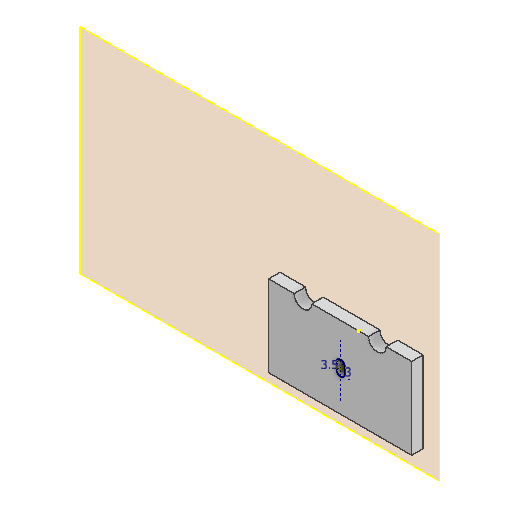
# Autodesk Inventor part: Cuvette Aligner 50mm
Saved by Autodesk Inventor 2025.1 (Build 291241020, 241B)
## iProperties
Created: 2024-09-23
Part Number: Cuvette Aligner 50mm
Material: Generic
Document SubType Name: Modeling
Designer: wayneslade
Density: 1 g/cm^3
Appearance: Default
Author: wayneslade
Autodesk Inventor part; units mm, degrees
ref_plane "YZ Plane" through (0, 0, 0) normal (1, 0, 0) x (0, 1, 0)
ref_plane "XZ Plane" through (0, 0, 0) normal (0, 1, 0) x (-1, 0, 0)
ref_plane "XY Plane" through (0, 0, 0) normal (0, 0, 1) x (1, 0, 0)
ref_plane "Work Plane1" through (0, 0, 0) normal (0, 0, 1) x (1, 0, 0)
sketch "Sketch1" plane through (0, 0, 0) normal (0, 0, 1) x (1, 0, 0)
  circle A0 centre (11.5562, -18) radius 2 construction
  line L0 (-53.1938, -16) -> (-53.1938, -30) construction
  arc A1 (-56.1938, -30) -> (-53.1938, -30) centre (-54.6938, -30) ccw construction
  line L1 (-56.1938, -30) -> (-56.1938, -16) construction
  arc A2 (-53.1938, -16) -> (-56.1938, -16) centre (-54.6938, -16) ccw construction
  line L2 (7.0562, -16) -> (7.0562, -30) construction
  arc A3 (4.0562, -30) -> (7.0562, -30) centre (5.5562, -30) ccw construction
  line L3 (4.0562, -30) -> (4.0562, -16) construction
  arc A4 (7.0562, -16) -> (4.0562, -16) centre (5.5562, -16) ccw construction
  line L4 (-13.1938, -16) -> (-13.1938, -30) construction
  arc A5 (-16.1938, -30) -> (-13.1938, -30) centre (-14.6938, -30) ccw construction
  line L5 (-16.1938, -30) -> (-16.1938, -16) construction
  arc A6 (-13.1938, -16) -> (-16.1938, -16) centre (-14.6938, -16) ccw construction
  arc A7 (19.0562, -16) -> (16.0562, -16) centre (17.5562, -16) ccw construction
  line L6 (19.0562, -16) -> (19.0562, -30) construction
  arc A8 (16.0562, -30) -> (19.0562, -30) centre (17.5562, -30) ccw construction
  line L7 (16.0562, -30) -> (16.0562, -16) construction
  line L8 (22.8064, -40) -> (22.8064, 45) construction
  line L9 (22.8064, 45) -> (-120, 45) construction
  line L10 (-120, 27.5563) -> (-120, 45) construction
  line L11 (-120, 27.5563) -> (-95.2035, 27.5563) construction
  arc A9 (-85.0841, 27.5563) -> (-95.2035, 27.5563) centre (-90.1438, 25.4) ccw construction
  line L12 (-85.0841, 27.5563) -> (17.8062, 27.5563) construction
  line L13 (17.8062, 27.5563) -> (17.8062, -11) construction
  line L14 (17.8062, -11) -> (-120, -11) construction
  line L15 (-120, -40) -> (-120, -11) construction
  line L16 (22.8064, -40) -> (-120, -40) construction
  circle A10 centre (-111.1938, -18) radius 2 construction
  circle A11 centre (-98.1938, -18) radius 2 construction
  circle A12 centre (-61.1938, -18) radius 2 construction
  circle A13 centre (-48.1938, -18) radius 2 construction
  circle A14 centre (-21.1938, -18) radius 2 construction
  circle A15 centre (-8.1938, -18) radius 2 construction
  circle A16 centre (-21.1938, 33.6563) radius 2 construction
  circle A17 centre (-8.1938, 33.6563) radius 2 construction
  circle A18 centre (-61.1938, 33.6563) radius 2 construction
  circle A19 centre (-48.1938, 33.6563) radius 2 construction
  circle A20 centre (-111.1938, 33.6563) radius 2 construction
  circle A21 centre (-98.1938, 33.6563) radius 2 construction
  circle A22 centre (-90.1438, -25.4) radius 5.5 construction
  circle A23 centre (7.8062, 0) radius 3.75 construction
  circle A24 centre (-24.6938, 0) radius 3.75 construction
  line L17 (22.8064, -35.5) -> (-39.6938, -35.5)
  line L18 (-39.6938, -35.5) -> (-39.6938, 0)
  line L19 (-39.6938, 0) -> (-28.5438, 0)
  line L20 (22.8064, 0) -> (22.8064, -35.5)
  line L21 (-34.6938, -11) -> (-34.6938, 11) construction
  arc A25 (3.9562, 0) -> (11.6562, 0) centre (7.8062, 0) ccw
  line L22 (11.6562, 0) -> (22.8064, 0)
  arc A26 (-28.5438, 0) -> (-20.8438, 0) centre (-24.6938, 0) ccw
  line L23 (-20.8438, 0) -> (3.9562, 0)
  point P0 (0, 0)
  point P1 (17.5562, -31.5)
  dimension "d0" = 5
  dimension "d1" = 0
  dimension "d2" = 0.1
  dimension "d3" = 0.1
  dimension "d4" = 4
  constraints: 12 end point, 5 point on circle, 4 parallel, 2 centre point, 2 coincident, 1 horizontal, 1 perpendicular, 1 point on line
  measures "d0" distance between parallel lines of L18 L21
  measures "d1" distance between parallel lines of L20 L8
  measures "d2" radial gap between concentric circles of A23 A25
  measures "d3" radial gap between concentric circles of A24 A26
  measures "d4" distance from line of L17 point (17.556, -31.5)
extrude "Main Body" add sketch "Sketch1" along normal blind 5
sketch "Sketch2" plane through (0, 0, 0) normal (0, 0, -1) x (-1, 0, 0)
  line L0 (16.1938, -30) -> (16.1938, -16) construction
  arc A0 (13.1938, -30) -> (16.1938, -30) centre (14.6938, -30) ccw construction
  line L1 (13.1938, -16) -> (13.1938, -30) construction
  arc A1 (16.1938, -16) -> (13.1938, -16) centre (14.6938, -16) ccw construction
  line L2 (16.1938, -30) -> (16.1938, -16) construction
  line L3 (-4.0562, -30) -> (-4.0562, -16) construction
  arc A2 (-7.0562, -30) -> (-4.0562, -30) centre (-5.5562, -30) ccw construction
  line L4 (-7.0562, -16) -> (-7.0562, -30) construction
  arc A3 (-4.0562, -16) -> (-7.0562, -16) centre (-5.5562, -16) ccw construction
  line L5 (-5.5562, -16) -> (-5.5562, -30) construction
  line L6 (14.6938, -16) -> (14.6938, -30) construction
  line L7 (-5.5562, -17) -> (-5.5562, -29) construction
  line L8 (-7.0062, -17) -> (-7.0062, -29)
  line L9 (-4.1062, -29) -> (-4.1062, -17)
  arc A4 (-4.1062, -17) -> (-7.0062, -17) centre (-5.5562, -17) ccw
  arc A5 (-7.0062, -29) -> (-4.1062, -29) centre (-5.5562, -29) ccw
  line L10 (14.6938, -17) -> (14.6938, -29) construction
  line L11 (13.2438, -17) -> (13.2438, -29)
  line L12 (16.1438, -29) -> (16.1438, -17)
  arc A6 (16.1438, -17) -> (13.2438, -17) centre (14.6938, -17) ccw
  arc A7 (13.2438, -29) -> (16.1438, -29) centre (14.6938, -29) ccw
  line L13 (-5.5562, -17) -> (14.6938, -17) construction
  line L14 (-5.5562, -29) -> (14.6938, -29) construction
  point P0 (0, 0)
  point P1 (-5.5562, -23)
  point P2 (14.6938, -23)
  dimension "d9" = 0.05
  dimension "d10" = 0.05
  dimension "d11" = 1
  dimension "d12" = 1
  constraints: 24 end point, 8 point on circle, 8 tangent, 4 centre point, 4 point on line, 2 horizontal, 2 midpoint, 2 parallel, 2 vertical
  measures "d9" distance between parallel lines of L4 L8
  measures "d10" distance between parallel lines of L11 L1
  measures "d11" distance of L7.start L5.start
  measures "d12" distance of L5.end L7.end
extrude "Alignment Tabs" add sketch "Sketch2" along normal blind 1.8
sketch "Sketch3" plane through (0, 0, 5) normal (0, 0, 1) x (1, 0, 0)
  circle A0 centre (-8.1938, -18) radius 2 construction
  line L0 (-8.1938, -31.3066) -> (-8.1938, -7.4741) construction
  line L1 (-8.1938, -16.5) -> (-8.1938, -19.5) construction
  line L2 (-6.4438, -16.5) -> (-6.4438, -19.5)
  line L3 (-9.9438, -19.5) -> (-9.9438, -16.5)
  arc A1 (-6.4438, -16.5) -> (-9.9438, -16.5) centre (-8.1938, -16.5) ccw
  arc A2 (-9.9438, -19.5) -> (-6.4438, -19.5) centre (-8.1938, -19.5) ccw
  point P0 (0, 0)
  dimension "d14" = 3.5
  dimension "d15" = 3
  constraints: 10 end point, 4 point on circle, 4 tangent, 2 centre point, 2 point on line, 1 midpoint, 1 parallel, 1 vertical
  measures "d14" distance between parallel lines of L3 L2
  measures "d15" distance of L1.start L1.end
extrude "Slot for Screw M3" cut sketch "Sketch3" against normal through all
equation "\"d3\" = d2"
equation "\"d10\" = d9"
equation "\"d12\" = d11"
body "Solid1"
